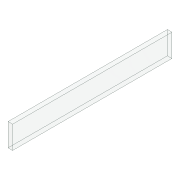
# Autodesk Inventor part: rail-210
Saved by Autodesk Inventor 2020 (Build 240168000, 168)
## iProperties
Created: 2021-06-22
Part Number: rail-210
Material: Generic
Document SubType Name: Modeling
Designer: Aidan Lee
Density: 1 g/cm^3
Appearance: Clear
Author: Aidan Lee
Autodesk Inventor part; units mm, degrees
ref_plane "YZ Plane" through (0, 0, 0) normal (1, 0, 0) x (0, 1, 0)
ref_plane "XZ Plane" through (0, 0, 0) normal (0, 1, 0) x (-1, 0, 0)
ref_plane "XY Plane" through (0, 0, 0) normal (0, 0, 1) x (1, 0, 0)
sketch "Sketch1" plane through (0, 0, 0) normal (1, 0, 0) x (0, 1, 0)
  line L0 (0, 0) -> (18, 0) construction
  line L1 (18, 0) -> (18, -390) construction
  line L2 (18, -390) -> (0, -390) construction
  line L3 (0, -390) -> (0, 0) construction
  line L4 (96, 0) -> (78, 0) construction
  line L5 (78, 0) -> (78, -210) construction
  line L6 (78, -210) -> (96, -210) construction
  line L7 (96, -210) -> (96, 0) construction
  line L8 (18, 0) -> (28, 0) construction
  line L9 (28, 0) -> (28, -210)
  line L10 (28, -210) -> (18, -210) construction
  line L11 (18, -210) -> (18, 0) construction
  circle A0 centre (53, -21.3494) radius 25 construction
  line L12 (28, 0) -> (13, 0)
  line L13 (13, 0) -> (13, -105)
  line L14 (13, -105) -> (28, -105)
  line L15 (28, 0) -> (35, 0)
  line L16 (35, 0) -> (35, -4)
  arc A1 (35, -4) -> (28, -11) centre (35, -11) ccw
  line L17 (28, -11) -> (28, -105)
  point P0 (20.5, -105)
  dimension "d6" = 50
  dimension "d0" = 18
  dimension "d1" = 210
  dimension "d2" = 18
  dimension "d3" = 60
  dimension "d4" = 390
  dimension "d5" = 10
  dimension "d7" = 5
  dimension "d11" = 7
  dimension "d12" = 4
  dimension "d13" = 7
  constraints: 36 end point, 6 parallel, 5 horizontal, 5 perpendicular, 3 vertical, 2 collinear, 2 midpoint, 2 point on circle, 1 centre point, 1 horizontal alignment, 1 tangent, 1 vertical alignment, 3 other
  measures "d0" distance of L0.start L0.end
  measures "d1" distance of L6.end L4.start
  measures "d2" distance of L4.start L4.end
  measures "d3" distance between parallel lines of L5 L1
  measures "d4" distance of L2.end L0.start
  measures "d5" distance between parallel lines of L1 L9
  measures "d7" distance between parallel lines of L1 L13
  measures "d11" distance of L8.end L15.end
  measures "d12" distance of L15.end L16.end
  measures "d13" radius of A1
extrude "Extrusion1" add sketch "Sketch1" along normal blind 3 contours L9 L14 L13 L12
body "Solid1"
